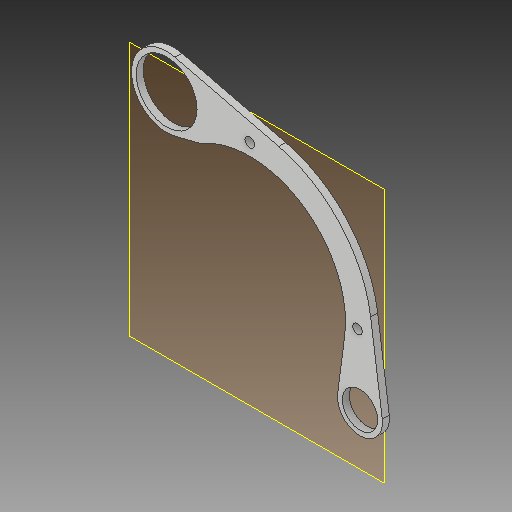
# Autodesk Inventor part: BackMotorPlate
Saved by Autodesk Inventor 2019.3 (Build 233278000, 278)
## iProperties
Created: 2018-12-14
Part Number: BackMotorPlate
Material: Generic
Document SubType Name: Modeling
Designer: eroldan
Density: 1 g/cm^3
Appearance: Default
Author: eroldan
Autodesk Inventor part; units mm, degrees
ref_plane "YZ Plane" through (0, 0, 0) normal (1, 0, 0) x (0, 1, 0)
ref_plane "XZ Plane" through (0, 0, 0) normal (0, 1, 0) x (-1, 0, 0)
ref_plane "XY Plane" through (0, 0, 0) normal (0, 0, 1) x (1, 0, 0)
ref_plane "Work Plane1" through (0, 0, 0) normal (0, 0, 1) x (1, 0, 0)
sketch "Sketch1" plane through (0, 0, 0) normal (0, 0, 1) x (1, 0, 0)
  circle A0 centre (0, 0) radius 63 construction
  circle A1 centre (-52.0914, 68.8152) radius 9 construction
  circle A2 centre (69.0649, -43.1304) radius 11.1125 projected
  arc A3 (55.0736, -41.2847) -> (83.0399, -41.1656) centre (69.0649, -43.1304) ccw
  circle A4 centre (-52.0914, 68.8152) radius 19.05
  arc A5 (-46.8467, 90.2323) -> (-46.6573, 47.4452) centre (-52.0914, 68.8152) ccw
  circle A6 centre (0, 0) radius 72.5 construction
  circle A7 centre (67.5, 0) radius 3 projected
  circle A8 centre (0, 67.5) radius 3 projected
  arc A9 (75.755, 10.6506) -> (18.1959, 74.3045) centre (0, 0) ccw
  line L0 (83.0399, -41.1656) -> (75.755, 10.6506)
  line L1 (18.1959, 74.3045) -> (-46.8467, 90.2323)
  arc A10 (59.4846, -7.8472) -> (-30.3603, 51.7518) centre (0, 0) ccw
  line L2 (-46.6573, 47.4452) -> (-31.3986, 51.3253)
  arc A11 (-31.3986, 51.3253) -> (-30.3603, 51.7518) centre (-32.3843, 55.202) ccw
  line L3 (55.0736, -41.2847) -> (59.4846, -7.8472)
  point P0 (0, 0)
  point P1 (73.2628, -22.0184)
  point P2 (80.1363, -20.5125)
  point P3 (-30.8402, 51.4673)
  dimension "d1" = 3
  dimension "d2" = 38.1
  dimension "d4" = 3
  dimension "d5" = 4
  dimension "d16" = 4
  dimension "d17" = 120
  constraints: 12 point on circle, 9 tangent, 8 end point, 6 centre point, 2 point on line, 1 coincident
  measures "d1" radial gap between concentric circles of A2 A3
  measures "d2" diameter of A4
  measures "d4" radial gap between concentric circles of A4 A5
  measures "d5" radial gap between concentric circles of A6 A9
  measures "d16" radius of A11
  measures "d17" diameter of A10
extrude "Extrusion1" add sketch "Sketch1" along normal blind 4.4
body "Solid1"
